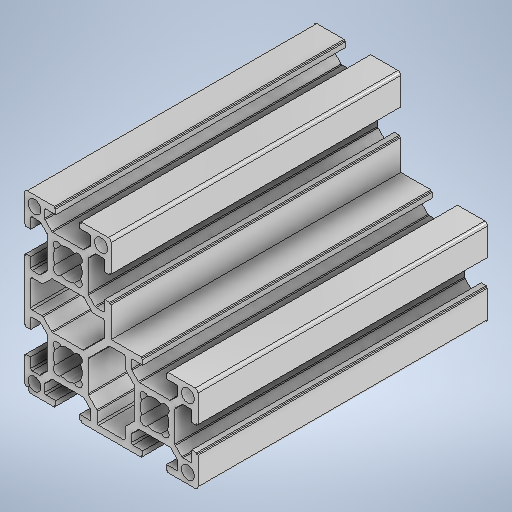
# Autodesk Inventor part: Perfil 60×60 L 8 rasgos_001
Saved by Autodesk Inventor 2026 (Build 300175000, 175)
## iProperties
Created: 2025-04-07
Part Number: Perfil 60×60 L 8 rasgos_001
Material: Aluminum 6061
Document SubType Name: Modeling
Designer: Carlos Dias
Density: 2.7 g/cm^3
Appearance: Aluminum - Polished
Author: Carlos Dias
Autodesk Inventor part; units mm, degrees
ref_plane "YZ Plane" through (0, 0, 0) normal (1, 0, 0) x (0, 1, 0)
ref_plane "XZ Plane" through (0, 0, 0) normal (0, 1, 0) x (-1, 0, 0)
ref_plane "XY Plane" through (0, 0, 0) normal (0, 0, 1) x (1, 0, 0)
sketch "Sketch1" plane through (0, 0, 0) normal (0, 0, 1) x (1, 0, 0)
  circle A0 centre (-15, 15) radius 5 construction
  circle A1 centre (-26.5, 3.5) radius 2.25 construction
  line L0 (0, 30) -> (-30, 0) construction
  line L1 (-30, 30) -> (0, 0) construction
  line L2 (-22, 22) -> (-22, 8) construction
  line L3 (-22, 22) -> (-8, 22) construction
  line L4 (-24.5556, 7) -> (-22, 9.5556)
  arc A2 (-24.909, 5.091) -> (-28.091, 1.909) centre (-26.5, 3.5) ccw
  line L5 (-27.8, 7) -> (-24.5556, 7)
  line L6 (-30, 0) -> (-30, 10.9) construction
  line L7 (-30, 10.9) -> (-27.8, 10.9) construction
  circle A3 centre (-18.5355, 18.5355) radius 1.5 construction
  arc A4 (-11.4645, 18.5355) -> (-17.3278, 19.4251) centre (-15, 15) ccw
  arc A5 (-17.3278, 19.4251) -> (-19.4251, 17.3278) centre (-18.5355, 18.5355) ccw
  line L8 (-27.8, 10.9) -> (-27.8, 7)
  arc A6 (-18.5355, 18.5355) -> (-19.4251, 12.6722) centre (-15, 15) ccw
  arc A7 (-19.4251, 12.6722) -> (-17.3278, 10.5749) centre (-18.5355, 11.4645) ccw
  arc A8 (-18.5355, 11.4645) -> (-12.6722, 10.5749) centre (-15, 15) ccw
  arc A9 (-12.6722, 10.5749) -> (-10.5749, 12.6722) centre (-11.4645, 11.4645) ccw
  arc A10 (-11.4645, 11.4645) -> (-10.5749, 17.3278) centre (-15, 15) ccw
  arc A11 (-10.5749, 17.3278) -> (-12.6722, 19.4251) centre (-11.4645, 18.5355) ccw
  line L9 (-30, 0) -> (-19.5962, 10.4038)
  line L10 (-24.5556, 23) -> (-22, 20.4444)
  line L11 (-27.8, 23) -> (-24.5556, 23)
  line L12 (-27.8, 23) -> (-27.8, 19.1)
  line L13 (-22, 20.4444) -> (-22, 9.5556)
  line L14 (-27.8, 19.1) -> (-30, 19.1) construction
  circle A12 centre (-15, 45) radius 5
  line L15 (-23.6444, 25.2) -> (-20.4444, 22)
  line L16 (-27.8, 25.2) -> (-23.6444, 25.2)
  line L17 (-30, 19.1) -> (-30, 40.9) construction
  line L18 (-2.2, 29.3556) -> (-9.5556, 22)
  line L19 (-20.4444, 22) -> (-9.5556, 22)
  circle A13 centre (-26.5, 56.5) radius 2.25
  line L20 (-30, 60) -> (-30, 49.1) construction
  line L21 (-30, 60) -> (0, 30) construction
  circle A14 centre (-18.5355, 48.5355) radius 1.5
  circle A15 centre (-18.5355, 41.4645) radius 1.5
  circle A16 centre (-11.4645, 41.4645) radius 1.5
  circle A17 centre (-11.4645, 48.5355) radius 1.5
  line L22 (-30, 40.9) -> (-27.8, 40.9) construction
  line L23 (-27.8, 40.9) -> (-27.8, 37)
  line L24 (-22, 52) -> (-22, 38) construction
  line L25 (0, 60) -> (-30, 30) construction
  line L26 (-22, 52) -> (-8, 52) construction
  line L27 (-8, 52) -> (-8, 38) construction
  line L28 (-8, 38) -> (-22, 38) construction
  line L29 (-22, 39.5556) -> (-24.5556, 37)
  line L30 (-20.4444, 38) -> (-23.6444, 34.8)
  line L31 (-24.5556, 37) -> (-27.8, 37)
  line L32 (-23.6444, 34.8) -> (-27.8, 34.8)
  line L33 (-27.8, 34.8) -> (-27.8, 25.2)
  line L34 (-30, 49.1) -> (-27.8, 49.1) construction
  line L35 (-27.8, 49.1) -> (-27.8, 53)
  line L36 (-27.8, 53) -> (-24.5556, 53)
  line L37 (-24.5556, 53) -> (-22, 50.4444)
  line L38 (-30, 60) -> (-19.1, 60) construction
  line L39 (-19.1, 60) -> (-19.1, 57.8) construction
  line L40 (-19.1, 57.8) -> (-23, 57.8)
  line L41 (-23, 57.8) -> (-23, 54.5556)
  line L42 (-23, 54.5556) -> (-20.4444, 52)
  line L43 (-22, 50.4444) -> (-22, 39.5556)
  line L44 (-7, 54.5556) -> (-9.5556, 52)
  line L45 (0, 60) -> (-10.9, 60) construction
  line L46 (-10.9, 60) -> (-10.9, 57.8) construction
  line L47 (-10.9, 57.8) -> (-7, 57.8)
  circle A18 centre (-3.5, 56.5) radius 2.25
  line L48 (-7, 57.8) -> (-7, 54.5556)
  line L49 (0, 60) -> (0, 49.1) construction
  line L50 (0, 49.1) -> (-2.2, 49.1) construction
  line L51 (-2.2, 49.1) -> (-2.2, 53)
  line L52 (-2.2, 53) -> (-5.4444, 53)
  line L53 (-5.4444, 53) -> (-8, 50.4444)
  line L54 (0, 40.9) -> (0, 30) construction
  line L55 (0, 40.9) -> (-2.2, 40.9) construction
  line L56 (-2.2, 40.9) -> (-2.2, 37)
  line L57 (-2.2, 37) -> (-5.4444, 37)
  line L58 (-5.4444, 37) -> (-8, 39.5556)
  line L59 (-9.5556, 38) -> (-6.3556, 34.8)
  line L60 (-6.3556, 34.8) -> (-2.2, 34.8)
  line L61 (-2.2, 34.8) -> (-2.2, 29.3556)
  line L62 (0, 30) -> (-10.4038, 19.5962)
  line L63 (-8, 50.4444) -> (-8, 39.5556)
  line L64 (-9.5556, 52) -> (-20.4444, 52)
  line L65 (-20.4444, 38) -> (-9.5556, 38)
  line L66 (-30, 10.9) -> (-29.5, 10.9) construction
  line L67 (-29.5, 10.9) -> (-29.5, 10.4)
  line L68 (-29.5, 10.4) -> (-30, 10.4)
  line L69 (-30, 10.4) -> (-30, 10.9) construction
  line L70 (-29.5, 10.9) -> (-27.8, 10.9)
  line L71 (-30, 10.4) -> (-30, 0)
  line L72 (-30, 19.1) -> (-29.5, 19.1) construction
  line L73 (-29.5, 19.1) -> (-29.5, 19.6)
  line L74 (-29.5, 19.6) -> (-30, 19.6)
  line L75 (-30, 19.6) -> (-30, 19.1) construction
  line L76 (-29.5, 19.1) -> (-27.8, 19.1)
  line L77 (-30, 40.9) -> (-29.5, 40.9) construction
  line L78 (-29.5, 40.9) -> (-29.5, 40.4)
  line L79 (-29.5, 40.4) -> (-30, 40.4)
  line L80 (-30, 40.4) -> (-30, 40.9) construction
  line L81 (-29.5, 40.9) -> (-27.8, 40.9)
  line L82 (-30, 40.4) -> (-30, 19.6)
  line L83 (-30, 49.1) -> (-29.5, 49.1) construction
  line L84 (-29.5, 49.1) -> (-29.5, 49.6)
  line L85 (-29.5, 49.6) -> (-30, 49.6)
  line L86 (-30, 49.6) -> (-30, 49.1) construction
  line L87 (-29.5, 49.1) -> (-27.8, 49.1)
  line L88 (-30, 60) -> (-30, 49.6)
  line L89 (-19.1, 60) -> (-19.6, 60) construction
  line L90 (-19.6, 60) -> (-19.6, 59.5)
  line L91 (-19.6, 59.5) -> (-19.1, 59.5)
  line L92 (-19.1, 59.5) -> (-19.1, 60) construction
  line L93 (-10.9, 60) -> (-10.4, 60) construction
  line L94 (-10.4, 60) -> (-10.4, 59.5)
  line L95 (-10.4, 59.5) -> (-10.9, 59.5)
  line L96 (-10.9, 59.5) -> (-10.9, 60) construction
  line L97 (0, 49.1) -> (-0.5, 49.1) construction
  line L98 (-0.5, 49.1) -> (-0.5, 49.6)
  line L99 (-0.5, 49.6) -> (0, 49.6)
  line L100 (0, 49.6) -> (0, 49.1) construction
  line L101 (0, 40.9) -> (-0.5, 40.9) construction
  line L102 (-0.5, 40.9) -> (-0.5, 40.4)
  line L103 (-0.5, 40.4) -> (0, 40.4)
  line L104 (0, 40.4) -> (0, 40.9) construction
  line L105 (0, 40.4) -> (0, 30)
  line L106 (-0.5, 40.9) -> (-2.2, 40.9)
  line L107 (-0.5, 49.1) -> (-2.2, 49.1)
  line L108 (0, 49.6) -> (0, 60)
  line L109 (0, 60) -> (-10.4, 60)
  line L110 (-10.9, 59.5) -> (-10.9, 57.8)
  line L111 (-19.1, 57.8) -> (-19.1, 59.5)
  line L112 (-19.6, 60) -> (-30, 60)
  point P0 (-26.1778, 23)
  point P1 (-10.5749, 47.3278)
  point P2 (-10.5749, 42.6722)
  point P3 (-12.6722, 40.5749)
  point P4 (-17.3278, 40.5749)
  point P5 (-19.4251, 42.6722)
  point P6 (-19.4251, 47.3278)
  point P7 (-17.3278, 49.4251)
  point P8 (-12.6722, 49.4251)
  point P9 (-24.909, 5.091)
  dimension "d23" = 10
  dimension "d0" = 10
  dimension "d1" = 15
  dimension "d2" = 15
  dimension "d3" = 4.5
  dimension "d4" = 26.5
  dimension "d7" = 8
  dimension "d8" = 30
  dimension "d9" = 1.1
  dimension "d10" = 1.25
  dimension "d11" = 4.1
  dimension "d12" = 2.2
  dimension "d13" = 3
  dimension "d20" = 360
  dimension "d22" = 1.1
  dimension "d24" = 30
  dimension "d25" = 2.2
  dimension "d26" = 4.1
  dimension "d27" = 1.1
  dimension "d28" = 4.5
  dimension "d29" = 53
  dimension "d30" = 60
  dimension "d31" = 3
  dimension "d34" = 360
  dimension "d36" = 8
  dimension "d38" = 1.1
  dimension "d39" = 4.5
  dimension "d40" = 0.5
  constraints: 224 end point, 51 equal length, 28 point on circle, 27 horizontal, 23 parallel, 18 centre point, 17 point on line, 17 vertical, 16 collinear, 13 perpendicular, 5 vertical alignment, 4 midpoint, 3 coincident, 3 concentric, 3 horizontal alignment, 53 other
  measures "d0" diameter of A0
  measures "d1" horizontal distance of point (0, 0) A0.centre
  measures "d2" horizontal distance of point (0, 0) A0.centre
  measures "d3" diameter of A1
  measures "d4" horizontal distance of point (0, 0) A1.centre
  measures "d7" distance from line of L6.start L2
  measures "d8" distance of point (0, 0) L6.start
  measures "d10" distance edge to line of A2 L5
  measures "d11" vertical distance of L6.end A0.centre
  measures "d12" distance of L6.end L7.end
  measures "d13" diameter of A3
  measures "d22" distance between parallel lines of L1 L10
  measures "d24" distance of point (-15, 45) A0.centre
  measures "d25" distance from line of point (-26.178, 23) L16
  measures "d26" vertical distance of point (-15, 45) L17.end
  measures "d28" diameter of A13
  measures "d29" distance of A1.centre A13.centre
  measures "d30" distance of L6.start L20.start
  measures "d31" diameter of A14
  measures "d36" distance from line of L17.end L24
  measures "d38" distance between parallel lines of L25 L29
  measures "d39" diameter of A18
  measures "d40" distance of L67.end L68.end
extrude "Extrusion1" add sketch "Sketch1" along normal mid plane 100 contours L4 L13 L10 L11 L12 L76 L73 L74 L82 L79 L78 L81 L23 L31 L29 L43 L37 L36 L35 L87 L84 L85 L88 L112 L90 L91 L111 L40 L41 L42 L64 L44 L48 L47 L110 L95 L94 L109 L108 L99 L98 L107 L51 L52 L53 L63 L58 L57 L56 L106 L102 L103 L105 L62 A11 A4 A5 A6 A7 L9 A2 L71 L68 L67 L70 L8 L5
fillet "Fillet1" radius 1 3 edges at (-30, 60, 0) (0, 60, 0) (-30, 0, 0)
fillet "Fillet2" radius 0.5 35 edges at (-22, 9.5556, 0) (-24.5556, 7, 0) (-9.5556, 22, 0) (-2.2, 29.3556, 0) (-2.2, 37, 0) (-22, 39.5556, 0) (-24.5556, 37, 0) (-9.5556, 52, 0) (-7, 54.5556, 0) (-27.8, 7, 0) (-20.4444, 22, 0) (-23.6444, 25.2, 0) (-27.8, 25.2, 0) (-8, 39.5556, 0) (-5.4444, 37, 0) (-20.4444, 52, 0) (-23, 54.5556, 0) (-27.8, 37, 0) (-27.8, 34.8, 0) (-23.6444, 34.8, 0) (-20.4444, 38, 0) (-9.5556, 38, 0) (-6.3556, 34.8, 0) (-27.8, 23, 0) (-24.5556, 23, 0) (-22, 20.4444, 0) (-22, 50.4444, 0) (-24.5556, 53, 0) (-2.2, 53, 0) (-7, 57.8, 0) (-2.2, 34.8, 0) (-23, 57.8, 0) (-27.8, 53, 0) (-8, 50.4444, 0) (-5.4444, 53, 0)
mirror "Mirror2" about plane through (-10.4038, 19.5962, 0) normal (0.7071068, -0.7071068, 0) of "Extrusion1", "Fillet1", "Fillet2"
equation "\"d23\" = d0"
equation "\"d2\" = d1"
equation "\"d22\" = d9"
equation "\"d24\" = d8"
equation "\"d25\" = d12"
equation "\"d26\" = d11"
equation "\"d27\" = d22"
equation "\"d28\" = d3"
equation "\"d31\" = d13"
equation "\"d36\" = d7"
equation "\"d38\" = d9"
equation "\"d39\" = d3"
body "Solid1"
